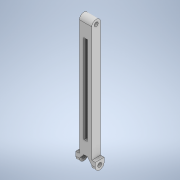
# Autodesk Inventor part: Rod
Saved by Autodesk Inventor 2022 (Build 260153000, 153)
## iProperties
Created: 2022-01-24
Part Number: Rod
Material: Generic
Document SubType Name: Modeling
Designer: alexa
Density: 1 g/cm^3
Appearance: Default
Author: alexa
Autodesk Inventor part; units mm, degrees
ref_plane "YZ Plane" through (0, 0, 0) normal (1, 0, 0) x (0, 1, 0)
ref_plane "XZ Plane" through (0, 0, 0) normal (0, 1, 0) x (-1, 0, 0)
ref_plane "XY Plane" through (0, 0, 0) normal (0, 0, 1) x (1, 0, 0)
sketch "Sketch1" plane through (0, 0, 0) normal (0, 0, 1) x (1, 0, 0)
  point P0 (0, 0)
sketch "Sketch2" plane through (0, 0, 0) normal (0, 0, 1) x (1, 0, 0)
  line L0 (0, 0) -> (0, 131)
  line L1 (0, 131) -> (14, 131)
  line L2 (14, 131) -> (14, 0)
  line L3 (0, 0) -> (-4, 0)
  line L4 (14, 0) -> (18, 0)
  line L5 (18, 0) -> (18, -10)
  line L6 (18, -10) -> (-4, -10)
  line L7 (-4, -10) -> (-4, 0)
  dimension "d0" = 14
  dimension "d17" = 4
  dimension "d18" = 10
  dimension "d19" = 4
  dimension "d38" = 131
  dimension "d39" = 131
  constraints: 16 end point, 5 perpendicular, 2 horizontal, 1 vertical
  measures "d0" distance of L0.start L2.end
  measures "d17" distance of L0.start L3.end
  measures "d18" distance of L4.end L5.end
  measures "d19" distance of L2.end L4.end
  measures "d38" distance of L0.start L0.end
  measures "d39" distance of L1.end L2.end
extrude "Extrusion1" add sketch "Sketch2" along normal blind 10
sketch "Sketch4" plane through (14, 0, 0) normal (1, 0, 0) x (0, 0, -1)
  line L0 (0, 131) -> (-10, 131) projected
  arc A0 (0, 131) -> (-10, 131) centre (-5, 131) ccw
  line L1 (0, 0) -> (-10, 0) projected
  arc A1 (-10, 0) -> (0, 0) centre (-5, 0) ccw
  dimension "d4" = 5
  dimension "d5" = 5
  constraints: 4 point on circle, 2 centre point
  measures "d4" radius of A1
  measures "d5" radius of A0
extrude "Extrusion2" add sketch "Sketch4" against normal blind 14 contours L0 A0
sketch "Sketch8" plane through (18, -10, 0) normal (1, 0, 0) x (0, 0, -1)
  circle A0 centre (-5, 5) radius 2.25
  line L0 (0, 0) -> (0, 10) projected
  line L1 (0, 0) -> (-10, 0) projected
  dimension "d21" = 4.5
  dimension "d22" = 5
  dimension "d23" = 5
  constraints: 1 centre point
  measures "d21" diameter of A0
  measures "d22" distance from line of L0 A0.centre
  measures "d23" distance from line of A0.centre L1
extrude "Extrusion6" cut sketch "Sketch8" against normal blind 22
fillet "Fillet1" radius 5 1 edges at (7, -10, 10)
fillet "Fillet2" radius 5 1 edges at (7, -10, 0)
sketch "Sketch10" plane through (14, 0, 10) normal (1, 0, 0) x (0, 0, -1)
  circle A0 centre (5, 131) radius 2.25
  line L0 (10, 0) -> (10, 131) projected
  arc A1 (10, 131) -> (0, 131) centre (5, 131) ccw projected
  dimension "d28" = 4.5
  dimension "d29" = 5
  dimension "d30" = 0
  constraints: 1 centre point
  measures "d28" diameter of A0
  measures "d29" distance from line of L0 A0.centre
  measures "d30" distance of A1.centre A0.centre
extrude "Extrusion7" cut sketch "Sketch10" against normal blind 14
sketch "Sketch11" plane through (0, 0, 0) normal (0, 0, -1) x (-1, 0, 0)
  line L0 (-4, 0) -> (-10, 0)
  line L1 (-10, 0) -> (-10, -10)
  line L2 (4, -10) -> (-18, -10) projected
  line L3 (-4, -10) -> (-4, 0)
  line L4 (-14, 0) -> (-14, 131) projected
  point P0 (0, 0)
  dimension "d33" = 4
  dimension "d34" = 4
  dimension "d35" = 6
  constraints: 6 end point, 2 point on line, 1 horizontal, 1 perpendicular
  measures "d33" distance of point (0, 0) L0.start
  measures "d34" distance from line of L4 L0.end
  measures "d35" distance of L1.end L3.start
extrude "Extrusion8" cut sketch "Sketch11" against normal blind 10
sketch "Sketch20" plane through (0, 0, 10) normal (0, 0, 1) x (1, 0, 0)
  line L0 (4, -5) -> (4, 0) projected
  line L1 (4, 0) -> (0, -5)
  line L2 (-4, -5) -> (4, -5) projected
  line L3 (4, -5) -> (4, -10) projected
  line L4 (0, -5) -> (4, -5)
  line L5 (4, 0) -> (4, -5)
  point P0 (0, 0)
  constraints: 6 end point, 2 perpendicular, 1 midpoint
extrude "Extrusion16" cut sketch "Sketch20" against normal blind 10
sketch "Sketch21" plane through (0, 0, 10) normal (0, 0, 1) x (1, 0, 0)
  line L0 (0, -5) -> (4, 0) projected
  line L1 (4, -5) -> (4, -10) projected
  line L2 (0, -5) -> (4, -5)
  line L3 (-4, -10) -> (4, -10) projected
  line L4 (4, -10) -> (0, -10)
  line L5 (-4, -5) -> (0, -5) projected
  line L6 (0, -5) -> (0, -10)
  line L7 (4, -5) -> (4, -10)
  point P0 (0, 0)
  constraints: 8 end point, 2 perpendicular, 1 midpoint, 1 parallel, 1 point on line
extrude "Extrusion17" cut sketch "Sketch21" against normal blind 10
sketch "Sketch22" plane through (0, 0, 10) normal (0, 0, 1) x (1, 0, 0)
  line L0 (10, -5) -> (10, 0) projected
  line L1 (10, 0) -> (14, -5)
  line L2 (10, -5) -> (18, -5) projected
  line L3 (10, 0) -> (10, -5)
  line L4 (10, -5) -> (14, -5)
  point P0 (0, 0)
  constraints: 6 end point, 1 midpoint, 1 perpendicular, 1 vertical
extrude "Extrusion18" cut sketch "Sketch22" against normal blind 10
sketch "Sketch23" plane through (0, 0, 10) normal (0, 0, 1) x (1, 0, 0)
  line L0 (10, -10) -> (10, -5) projected
  line L1 (18, -5) -> (14, -5) projected
  line L2 (10, -5) -> (14, -5)
  line L3 (14, -5) -> (14, -10)
  line L4 (10, -10) -> (18, -10) projected
  line L5 (10, -5) -> (10, -10)
  line L6 (10, -10) -> (14, -10)
  point P0 (0, 0)
  constraints: 8 end point, 1 horizontal, 1 midpoint, 1 perpendicular, 1 vertical
extrude "Extrusion19" cut sketch "Sketch23" against normal blind 10
sketch "Sketch24" plane through (0, 0, 10) normal (0, 0, 1) x (1, 0, 0)
  line L0 (4, 0) -> (10, 0) projected
  line L1 (4, 0) -> (4.8, 1)
  line L2 (0, -5) -> (4, 0) projected
  line L3 (4.8, 1) -> (9.2, 1)
  line L4 (14, -5) -> (10, 0) projected
  line L5 (9.2, 1) -> (10, 0)
  point P0 (0, 0)
  dimension "d66" = 1
  constraints: 6 end point, 2 collinear, 1 horizontal
  measures "d66" vertical distance of L0.start L1.end
extrude "Extrusion20" cut sketch "Sketch24" against normal blind 10
sketch "Sketch25" plane through (0, 0, 10) normal (0, 0, 1) x (1, 0, 0)
  line L0 (5, 116) -> (9, 116)
  line L1 (9, 116) -> (9, 16)
  line L2 (9, 16) -> (5, 16)
  line L3 (5, 16) -> (5, 116)
  line L4 (14, 0) -> (14, 131) projected
  line L5 (14, 131) -> (0, 131) projected
  line L6 (4.8, 1) -> (9.2, 1) projected
  line L7 (0, 131) -> (0, 0) projected
  dimension "d82" = 5
  dimension "d84" = 4
  dimension "d85" = 100
  dimension "d86" = 15
  constraints: 8 end point, 2 perpendicular
  measures "d82" distance between parallel lines of L7 L3
  measures "d84" distance of L0.start L0.end
  measures "d85" distance of L0.end L1.end
  measures "d86" distance between parallel lines of L0 L5
extrude "Extrusion21" cut sketch "Sketch25" against normal blind 10
body "Solid1"
